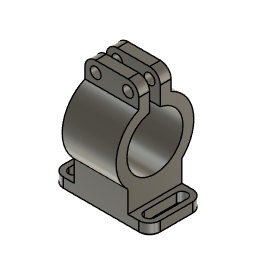
Motor Clamp MK 2 v3 (Autodesk Fusion 360 design; units mm, degrees)
Autodesk Fusion 360 part; units mm, degrees
sketch "Sketch1" plane through (0, 0, 0) normal (0, 0, 1) x (1, 0, 0)
  line L0 (22.5, 12.5) -> (-22.5, 12.5)
  line L1 (-22.5, 12.5) -> (-22.5, -12.5)
  line L2 (-22.5, -12.5) -> (22.5, -12.5)
  line L3 (22.5, -12.5) -> (22.5, 12.5)
  line L4 (22.5, 12.5) -> (-22.5, -12.5) construction
  line L5 (-22.5, 12.5) -> (22.5, -12.5) construction
  line L6 (-17.5, 12.5) -> (-17.5, -12.5) construction
  line L7 (0, -12.5) -> (0, 12.5) construction
  line L8 (-22.5, 0) -> (22.5, 0) construction
  line L9 (-20, 7.5) -> (-20, -7.5)
  line L10 (-15, -7.5) -> (-15, 7.5)
  arc A0 (-15, 7.5) -> (-20, 7.5) centre (-17.5, 7.5) ccw
  arc A1 (-20, -7.5) -> (-17.5, -5) centre (-17.5, -7.5) ccw
  line L11 (12.5, 12.5) -> (-12.5, 12.5)
  line L12 (-12.5, 12.5) -> (-12.5, -12.5)
  line L13 (-12.5, -12.5) -> (12.5, -12.5)
  line L14 (12.5, -12.5) -> (12.5, 12.5)
  line L15 (12.5, 12.5) -> (-12.5, -12.5) construction
  line L16 (-12.5, 12.5) -> (12.5, -12.5) construction
  arc A2 (20, 7.5) -> (15, 7.5) centre (17.5, 7.5) ccw
  line L17 (15, -7.5) -> (15, 7.5)
  line L18 (20, 7.5) -> (20, -7.5)
  arc A3 (17.5, -5) -> (20, -7.5) centre (17.5, -7.5) ccw
  dimension "d1" = 45
  dimension "d2" = 25
  dimension "d3" = 5
  dimension "d4" = 5
  dimension "d5" = 5
  dimension "d6" = 15
  dimension "d7" = 25
  dimension "d8" = 25
  constraint horizontal L0
  constraint perpendicular L0 L1
  constraint parallel L0 L2
  constraint parallel L1 L3
  constraint coincident L4 origin
  constraint coincident L5 origin
  constraint coincident L0 L6.start
  constraint coincident L2 L6.end
  constraint perpendicular L2 L6
  constraint midpoint L2 L7.start
  constraint midpoint L0 L7.end
  constraint coincident L6 A0.centre
  constraint coincident L6 A1.centre
  constraint midpoint L1 L8.start
  constraint midpoint L3 L8.end
  constraint symmetric L8 A0 A1
  constraint tangent L9 A1
  constraint coincident L10.start A1
  constraint tangent L10 A0
  constraint perpendicular L8 L10
  constraint tangent L9 A0
  constraint coincident L6 A1.end
  constraint horizontal L11
  constraint perpendicular L11 L12
  constraint parallel L11 L13
  constraint parallel L12 L14
  constraint coincident L15 origin
  constraint coincident L16 origin
  constraint symmetric L7 L9.start A2.start
  constraint symmetric L7 L9.end L18.end
  constraint symmetric L7 L10.start L17.start
  constraint symmetric L7 L10.end A2.end
  constraint symmetric L7 A0 A2
  constraint symmetric L7 A1.end A3.start
  constraint symmetric L7 A1 A3
  measures "d1" distance of L1.end L2.end L7
  measures "d2" distance of L0.end L1.end L7
  measures "d3" distance of L1 L6
  measures "d4" diameter of A0
  measures "d5" diameter of A1
  measures "d6" distance of A0.centre A1.centre
  measures "d7" distance of L12.end L13.end
  measures "d8" distance of L11.end L12.end
extrude "Extrude1" add sketch "Sketch1" along normal blind 5 contours L0 L2 L3 L14 | L0 L1 L2 L12 makes body 1 at (13.3333, -2.5, 0) makes body 2 at (-13.3333, -2.5, 0)
extrude "Extrude2" add sketch "Sketch1" along normal blind 15 contours L0 L2 L11 L12 L13 L14 bodies 1 2
sketch "Sketch2" plane through (12.5, 0, 0) normal (1, 0, 0) x (0, 1, 0)
  line L0 (-12.5, 5) -> (12.5, 5)
  line L1 (12.5, 5) -> (12.5, 15)
  line L2 (12.5, 15) -> (-12.5, 15)
  line L3 (-12.5, 15) -> (-12.5, 5)
  line L4 (-12.5, 15) -> (12.5, 15)
  circle A0 centre (0, 28) radius 13
  circle A1 centre (0, 28) radius 18.0347
  line L5 (0, 28) -> (0, 59) construction
  line L6 (-2.5, 40.7574) -> (-2.5, 54.4012)
  line L7 (2.5, 40.7574) -> (2.5, 54.4012)
  line L8 (-7.5, 38.6184) -> (-7.5, 54.4012)
  line L9 (7.5, 38.6184) -> (7.5, 54.4012)
  line L10 (-7.5, 54.4012) -> (-2.5, 54.4012)
  line L11 (2.5, 54.4012) -> (7.5, 54.4012)
  point P0 (0, 15)
  point P1 (7.5, 44.4012)
  dimension "d13" = 26
  dimension "d14" = 36.0694
  dimension "d15" = 5
  dimension "d17" = 5
  dimension "d18" = 5
  dimension "d20" = 10
  constraint midpoint L4 P0
  constraint vertical P0 A0.centre
  constraint coincident P0 A0
  constraint concentric A0 A1
  constraint coincident L1.end A1
  constraint coincident A0.centre A1.centre
  constraint vertical L5
  constraint coincident A0 L6.start
  constraint vertical L6
  constraint coincident A0 L7.start
  constraint vertical L7
  constraint symmetric L5 L6 L7
  constraint coincident A0 L8.start
  constraint parallel L6 L8
  constraint coincident A0 L9.start
  constraint vertical L9
  constraint horizontal L6.end L8.end
  constraint horizontal L7.end L9.end
  constraint horizontal L6.end L7.end
  constraint coincident L9 P1
  constraint coincident A1 P1
  measures "d13" diameter of A0
  measures "d14" diameter of A1
  measures "d15" distance of L6 L7
  measures "d17" distance of L6 L8
  measures "d18" distance of L7 L9
  measures "d20" distance of L9.end P1
extrude "Extrude3" add sketch "Sketch2" against normal blind 25 contours L2 L4 A0 A1 L8 | L2 L4 A0 A1 L9 | A1 L6 L8 L10 | A0 A1 L6 L8 | A0 A1 L7 L9 | A1 L7 L9 L11 bodies 1
sketch "Sketch3" plane through (0, -7.5, 0) normal (0, -1, 0) x (1, 0, 0)
  line L0 (12.5, 44.4012) -> (12.5, 54.4012)
  line L1 (12.5, 54.4012) -> (-12.5, 54.4012)
  line L2 (-12.5, 54.4012) -> (-12.5, 44.4012)
  line L3 (-12.5, 44.4012) -> (12.5, 44.4012)
  line L4 (0, 54.4012) -> (0, 44.4012) construction
  line L5 (-12.5, 49.4012) -> (12.5, 49.4012) construction
  circle A0 centre (-7.5, 49.4012) radius 2.5
  circle A1 centre (7.5, 49.4012) radius 2.5
  dimension "d23" = 5
  dimension "d24" = 5
  dimension "d25" = 15
  constraint midpoint L1 L4.start
  constraint midpoint L3 L4.end
  constraint midpoint L2 L5.start
  constraint midpoint L0 L5.end
  constraint coincident L5 A0.centre
  constraint coincident L5 A1.centre
  constraint symmetric L4 A0 A1
  measures "d23" diameter of A0
  measures "d24" diameter of A1
  measures "d25" distance of A0.centre A1.centre
extrude "Extrude4" cut sketch "Sketch3" against normal through all contours A0 | A1 bodies 1
fillet "Fillet1" radius 5 4 edges at (-22.5, 12.5, 2.5) (-22.5, -12.5, 2.5) (22.5, 12.5, 2.5) (22.5, -12.5, 2.5) on bodies 1
fillet "Fillet2" radius 5 4 edges at (12.5, -5, 54.4012) (12.5, 5, 54.4012) (-12.5, -5, 54.4012) (-12.5, 5, 54.4012) on bodies 1
chamfer "Chamfer1" distance 0.5 angle 45 1 faces at (-5, -2.5, 0) on bodies 1
